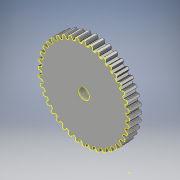
# Autodesk Inventor part: Engranaje_V_G_1
Saved by Autodesk Inventor 2017 (Build 210142000, 142)
## iProperties
Created: 2016-10-02
Part Number: Engranaje_V_G_1
Material: Generic
Document SubType Name: Modeling
Designer: CASA
Density: 1 g/cm^3
Appearance: Default
Author: CASA
Autodesk Inventor part; units mm, degrees
(part 1 of 3)
ref_plane "YZ Plane" through (0, 0, 0) normal (1, 0, 0) x (0, 1, 0)
ref_plane "XZ Plane" through (0, 0, 0) normal (0, 1, 0) x (-1, 0, 0)
ref_plane "XY Plane" through (0, 0, 0) normal (0, 0, 1) x (1, 0, 0)
sketch "Sketch1" plane through (0, 0, 0) normal (0, 1, 0) x (-1, 0, 0)
  line L0 (1.2517, 1.1017) -> (1.2466, 1.0629)
  line L1 (1.2466, 1.0629) -> (1.2316, 1.0267)
  line L2 (1.2316, 1.0267) -> (1.2078, 0.9957)
  line L3 (1.2078, 0.9957) -> (1.1767, 0.9718)
  line L4 (1.1767, 0.9718) -> (1.1405, 0.9568)
  line L5 (1.1405, 0.9568) -> (1.1017, 0.9517)
  line L6 (1.1017, 0.9517) -> (1.0629, 0.9568)
  line L7 (1.0629, 0.9568) -> (1.0267, 0.9718)
  line L8 (1.0267, 0.9718) -> (0.9956, 0.9956)
  line L9 (0.9956, 0.9956) -> (0.9718, 1.0267)
  line L10 (0.9718, 1.0267) -> (0.9568, 1.0629)
  line L11 (0.9568, 1.0629) -> (0.9517, 1.1017)
  line L12 (0.9517, 1.1017) -> (0.9568, 1.1405)
  line L13 (0.9568, 1.1405) -> (0.9718, 1.1767)
  line L14 (0.9718, 1.1767) -> (0.9956, 1.2078)
  line L15 (0.9956, 1.2078) -> (1.0267, 1.2316)
  line L16 (1.0267, 1.2316) -> (1.0629, 1.2466)
  line L17 (1.0629, 1.2466) -> (1.1017, 1.2517)
  line L18 (1.1017, 1.2517) -> (1.1405, 1.2466)
  line L19 (1.1405, 1.2466) -> (1.1767, 1.2316)
  line L20 (1.1767, 1.2316) -> (1.2078, 1.2078)
  line L21 (1.2078, 1.2078) -> (1.2316, 1.1767)
  line L22 (1.2316, 1.1767) -> (1.2466, 1.1405)
  line L23 (1.2466, 1.1405) -> (1.2517, 1.1017)
  line L24 (2.1254, 1.1532) -> (2.1288, 1.1525)
  line L25 (2.1288, 1.1525) -> (2.1355, 1.1511)
  line L26 (2.1355, 1.1511) -> (2.149, 1.1477)
  line L27 (2.149, 1.1477) -> (2.1625, 1.1437)
  line L28 (2.1625, 1.1437) -> (2.1761, 1.139)
  line L29 (2.1761, 1.139) -> (2.1896, 1.1339)
  line L30 (2.1896, 1.1339) -> (2.2031, 1.1282)
  line L31 (2.2031, 1.1282) -> (2.2031, 1.0756)
  line L32 (2.2031, 1.0756) -> (2.1896, 1.0699)
  line L33 (2.1896, 1.0699) -> (2.1761, 1.0647)
  line L34 (2.1761, 1.0647) -> (2.1626, 1.0601)
  line L35 (2.1626, 1.0601) -> (2.1491, 1.0561)
  line L36 (2.1491, 1.0561) -> (2.1356, 1.0527)
  line L37 (2.1356, 1.0527) -> (2.1288, 1.0513)
  line L38 (2.1288, 1.0513) -> (2.1254, 1.0506)
  line L39 (2.1254, 1.0506) -> (2.1221, 1.05)
  line L40 (2.1221, 1.05) -> (2.1176, 0.9935)
  line L41 (2.1176, 0.9935) -> (2.1209, 0.9923)
  line L42 (2.1209, 0.9923) -> (2.1241, 0.9912)
  line L43 (2.1241, 0.9912) -> (2.1305, 0.9887)
  line L44 (2.1305, 0.9887) -> (2.1433, 0.9832)
  line L45 (2.1433, 0.9832) -> (2.156, 0.9772)
  line L46 (2.156, 0.9772) -> (2.1687, 0.9705)
  line L47 (2.1687, 0.9705) -> (2.1812, 0.9633)
  line L48 (2.1812, 0.9633) -> (2.1936, 0.9556)
  line L49 (2.1936, 0.9556) -> (2.1854, 0.9035)
  line L50 (2.1854, 0.9035) -> (2.1712, 0.9)
  line L51 (2.1712, 0.9) -> (2.1571, 0.897)
  line L52 (2.1571, 0.897) -> (2.143, 0.8945)
  line L53 (2.143, 0.8945) -> (2.129, 0.8927)
  line L54 (2.129, 0.8927) -> (2.1151, 0.8914)
  line L55 (2.1151, 0.8914) -> (2.1083, 0.8911)
  line L56 (2.1083, 0.8911) -> (2.1048, 0.891)
  line L57 (2.1048, 0.891) -> (2.1014, 0.8909)
  line L58 (2.1014, 0.8909) -> (2.0882, 0.8357)
  line L59 (2.0882, 0.8357) -> (2.0912, 0.8341)
  line L60 (2.0912, 0.8341) -> (2.0942, 0.8325)
  line L61 (2.0942, 0.8325) -> (2.1002, 0.829)
  line L62 (2.1002, 0.829) -> (2.112, 0.8216)
  line L63 (2.112, 0.8216) -> (2.1236, 0.8136)
  line L64 (2.1236, 0.8136) -> (2.135, 0.8051)
  line L65 (2.135, 0.8051) -> (2.1462, 0.796)
  line L66 (2.1462, 0.796) -> (2.1573, 0.7864)
  line L67 (2.1573, 0.7864) -> (2.1411, 0.7364)
  line L68 (2.1411, 0.7364) -> (2.1265, 0.7351)
  line L69 (2.1265, 0.7351) -> (2.112, 0.7344)
  line L70 (2.112, 0.7344) -> (2.0978, 0.7342)
  line L71 (2.0978, 0.7342) -> (2.0837, 0.7345)
  line L72 (2.0837, 0.7345) -> (2.0698, 0.7355)
  line L73 (2.0698, 0.7355) -> (2.0629, 0.7362)
  line L74 (2.0629, 0.7362) -> (2.0595, 0.7366)
  line L75 (2.0595, 0.7366) -> (2.0561, 0.7371)
  line L76 (2.0561, 0.7371) -> (2.0344, 0.6847)
  line L77 (2.0344, 0.6847) -> (2.0371, 0.6826)
  line L78 (2.0371, 0.6826) -> (2.0398, 0.6805)
  line L79 (2.0398, 0.6805) -> (2.0452, 0.6762)
  line L80 (2.0452, 0.6762) -> (2.0557, 0.667)
  line L81 (2.0557, 0.667) -> (2.0659, 0.6573)
  line L82 (2.0659, 0.6573) -> (2.0759, 0.6471)
  line L83 (2.0759, 0.6471) -> (2.0856, 0.6363)
  line L84 (2.0856, 0.6363) -> (2.095, 0.6252)
  line L85 (2.095, 0.6252) -> (2.0711, 0.5783)
  line L86 (2.0711, 0.5783) -> (2.0565, 0.5794)
  line L87 (2.0565, 0.5794) -> (2.0421, 0.5809)
  line L88 (2.0421, 0.5809) -> (2.028, 0.5829)
  line L89 (2.028, 0.5829) -> (2.0141, 0.5855)
  line L90 (2.0141, 0.5855) -> (2.0006, 0.5886)
  line L91 (2.0006, 0.5886) -> (1.9939, 0.5903)
  line L92 (1.9939, 0.5903) -> (1.9906, 0.5913)
  line L93 (1.9906, 0.5913) -> (1.9873, 0.5923)
  line L94 (1.9873, 0.5923) -> (1.9577, 0.5439)
  line L95 (1.9577, 0.5439) -> (1.9601, 0.5415)
  line L96 (1.9601, 0.5415) -> (1.9624, 0.5389)
  line L97 (1.9624, 0.5389) -> (1.967, 0.5338)
  line L98 (1.967, 0.5338) -> (1.976, 0.5231)
  line L99 (1.976, 0.5231) -> (1.9845, 0.5119)
  line L100 (1.9845, 0.5119) -> (1.9928, 0.5003)
  line L101 (1.9928, 0.5003) -> (2.0006, 0.4882)
  line L102 (2.0006, 0.4882) -> (2.0082, 0.4756)
  line L103 (2.0082, 0.4756) -> (1.9773, 0.4331)
  line L104 (1.9773, 0.4331) -> (1.9631, 0.4364)
  line L105 (1.9631, 0.4364) -> (1.9491, 0.4402)
  line L106 (1.9491, 0.4402) -> (1.9355, 0.4444)
  line L107 (1.9355, 0.4444) -> (1.9221, 0.4491)
  line L108 (1.9221, 0.4491) -> (1.9092, 0.4543)
  line L109 (1.9092, 0.4543) -> (1.9029, 0.4571)
  line L110 (1.9029, 0.4571) -> (1.8998, 0.4585)
  line L111 (1.8998, 0.4585) -> (1.8968, 0.46)
  line L112 (1.8968, 0.46) -> (1.8599, 0.4169)
  line L113 (1.8599, 0.4169) -> (1.8619, 0.4141)
  line L114 (1.8619, 0.4141) -> (1.8638, 0.4112)
  line L115 (1.8638, 0.4112) -> (1.8675, 0.4054)
  line L116 (1.8675, 0.4054) -> (1.8747, 0.3935)
  line L117 (1.8747, 0.3935) -> (1.8814, 0.3811)
  line L118 (1.8814, 0.3811) -> (1.8877, 0.3683)
  line L119 (1.8877, 0.3683) -> (1.8936, 0.3551)
  line L120 (1.8936, 0.3551) -> (1.8991, 0.3415)
  line L121 (1.8991, 0.3415) -> (1.8619, 0.3043)
  line L122 (1.8619, 0.3043) -> (1.8484, 0.3099)
  line L123 (1.8484, 0.3099) -> (1.8352, 0.3158)
  line L124 (1.8352, 0.3158) -> (1.8224, 0.3221)
  line L125 (1.8224, 0.3221) -> (1.81, 0.3288)
  line L126 (1.81, 0.3288) -> (1.798, 0.3359)
  line L127 (1.798, 0.3359) -> (1.7922, 0.3397)
  line L128 (1.7922, 0.3397) -> (1.7894, 0.3416)
  line L129 (1.7894, 0.3416) -> (1.7866, 0.3436)
  line L130 (1.7866, 0.3436) -> (1.7434, 0.3067)
  line L131 (1.7434, 0.3067) -> (1.7449, 0.3036)
  line L132 (1.7449, 0.3036) -> (1.7464, 0.3005)
  line L133 (1.7464, 0.3005) -> (1.7492, 0.2942)
  line L134 (1.7492, 0.2942) -> (1.7544, 0.2813)
  line L135 (1.7544, 0.2813) -> (1.7591, 0.268)
  line L136 (1.7591, 0.268) -> (1.7633, 0.2544)
  line L137 (1.7633, 0.2544) -> (1.7671, 0.2404)
  line L138 (1.7671, 0.2404) -> (1.7704, 0.2261)
  line L139 (1.7704, 0.2261) -> (1.7278, 0.1952)
  line L140 (1.7278, 0.1952) -> (1.7153, 0.2028)
  line L141 (1.7153, 0.2028) -> (1.7032, 0.2107)
  line L142 (1.7032, 0.2107) -> (1.6915, 0.2189)
  line L143 (1.6915, 0.2189) -> (1.6803, 0.2275)
  line L144 (1.6803, 0.2275) -> (1.6696, 0.2364)
  line L145 (1.6696, 0.2364) -> (1.6645, 0.241)
  line L146 (1.6645, 0.241) -> (1.662, 0.2434)
  line L147 (1.662, 0.2434) -> (1.6596, 0.2458)
  line L148 (1.6596, 0.2458) -> (1.6112, 0.2161)
  line L149 (1.6112, 0.2161) -> (1.6122, 0.2128)
  line L150 (1.6122, 0.2128) -> (1.6131, 0.2095)
  line L151 (1.6131, 0.2095) -> (1.6149, 0.2029)
  line L152 (1.6149, 0.2029) -> (1.618, 0.1893)
  line L153 (1.618, 0.1893) -> (1.6206, 0.1754)
  line L154 (1.6206, 0.1754) -> (1.6226, 0.1613)
  line L155 (1.6226, 0.1613) -> (1.6241, 0.1469)
  line L156 (1.6241, 0.1469) -> (1.6252, 0.1323)
  line L157 (1.6252, 0.1323) -> (1.5783, 0.1084)
  line L158 (1.5783, 0.1084) -> (1.5671, 0.1179)
  line L159 (1.5671, 0.1179) -> (1.5564, 0.1276)
  line L160 (1.5564, 0.1276) -> (1.5462, 0.1375)
  line L161 (1.5462, 0.1375) -> (1.5364, 0.1477)
  line L162 (1.5364, 0.1477) -> (1.5273, 0.1582)
  line L163 (1.5273, 0.1582) -> (1.5229, 0.1636)
  line L164 (1.5229, 0.1636) -> (1.5208, 0.1663)
  line L165 (1.5208, 0.1663) -> (1.5188, 0.169)
  line L166 (1.5188, 0.169) -> (1.4663, 0.1473)
  line L167 (1.4663, 0.1473) -> (1.4668, 0.1439)
  line L168 (1.4668, 0.1439) -> (1.4673, 0.1405)
  line L169 (1.4673, 0.1405) -> (1.468, 0.1337)
  line L170 (1.468, 0.1337) -> (1.4689, 0.1198)
  line L171 (1.4689, 0.1198) -> (1.4693, 0.1057)
  line L172 (1.4693, 0.1057) -> (1.469, 0.0914)
  line L173 (1.469, 0.0914) -> (1.4683, 0.077)
  line L174 (1.4683, 0.077) -> (1.4671, 0.0624)
  line L175 (1.4671, 0.0624) -> (1.4171, 0.0461)
  line L176 (1.4171, 0.0461) -> (1.4075, 0.0572)
  line L177 (1.4075, 0.0572) -> (1.3984, 0.0684)
  line L178 (1.3984, 0.0684) -> (1.3898, 0.0799)
  line L179 (1.3898, 0.0799) -> (1.3818, 0.0915)
  line L180 (1.3818, 0.0915) -> (1.3744, 0.1033)
  line L181 (1.3744, 0.1033) -> (1.371, 0.1092)
  line L182 (1.371, 0.1092) -> (1.3693, 0.1123)
  line L183 (1.3693, 0.1123) -> (1.3677, 0.1153)
  line L184 (1.3677, 0.1153) -> (1.3126, 0.102)
  line L185 (1.3126, 0.102) -> (1.3125, 0.0986)
  line L186 (1.3125, 0.0986) -> (1.3124, 0.0952)
  line L187 (1.3124, 0.0952) -> (1.312, 0.0883)
  line L188 (1.312, 0.0883) -> (1.3108, 0.0744)
  line L189 (1.3108, 0.0744) -> (1.3089, 0.0604)
  line L190 (1.3089, 0.0604) -> (1.3065, 0.0464)
  line L191 (1.3065, 0.0464) -> (1.3035, 0.0322)
  line L192 (1.3035, 0.0322) -> (1.3, 0.018)
  line L193 (1.3, 0.018) -> (1.248, 0.0098)
  line L194 (1.248, 0.0098) -> (1.2403, 0.0222)
  line L195 (1.2403, 0.0222) -> (1.2331, 0.0348)
  line L196 (1.2331, 0.0348) -> (1.2264, 0.0474)
  line L197 (1.2264, 0.0474) -> (1.2203, 0.0601)
  line L198 (1.2203, 0.0601) -> (1.2149, 0.0729)
  line L199 (1.2149, 0.0729) -> (1.2124, 0.0793)
  line L200 (1.2124, 0.0793) -> (1.2112, 0.0826)
  line L201 (1.2112, 0.0826) -> (1.2101, 0.0858)
  line L202 (1.2101, 0.0858) -> (1.1536, 0.0814)
  line L203 (1.1536, 0.0814) -> (1.153, 0.078)
  line L204 (1.153, 0.078) -> (1.1523, 0.0746)
  line L205 (1.1523, 0.0746) -> (1.1509, 0.0679)
  line L206 (1.1509, 0.0679) -> (1.1475, 0.0544)
  line L207 (1.1475, 0.0544) -> (1.1435, 0.0409)
  line L208 (1.1435, 0.0409) -> (1.1389, 0.0273)
  line L209 (1.1389, 0.0273) -> (1.1337, 0.0138)
  line L210 (1.1337, 0.0138) -> (1.128, 0.0003)
  line L211 (1.128, 0.0003) -> (1.0754, 0.0003)
  line L212 (1.0754, 0.0003) -> (1.0697, 0.0138)
  line L213 (1.0697, 0.0138) -> (1.0646, 0.0273)
  line L214 (1.0646, 0.0273) -> (1.06, 0.0409)
  line L215 (1.06, 0.0409) -> (1.0559, 0.0544)
  line L216 (1.0559, 0.0544) -> (1.0525, 0.0679)
  line L217 (1.0525, 0.0679) -> (1.0511, 0.0746)
  line L218 (1.0511, 0.0746) -> (1.0505, 0.078)
  line L219 (1.0505, 0.078) -> (1.0499, 0.0814)
  line L220 (1.0499, 0.0814) -> (0.9933, 0.0858)
  line L221 (0.9933, 0.0858) -> (0.9922, 0.0826)
  line L222 (0.9922, 0.0826) -> (0.991, 0.0793)
  line L223 (0.991, 0.0793) -> (0.9886, 0.0729)
  line L224 (0.9886, 0.0729) -> (0.9831, 0.0601)
  line L225 (0.9831, 0.0601) -> (0.977, 0.0474)
  line L226 (0.977, 0.0474) -> (0.9703, 0.0348)
  line L227 (0.9703, 0.0348) -> (0.9631, 0.0222)
  line L228 (0.9631, 0.0222) -> (0.9554, 0.0098)
  line L229 (0.9554, 0.0098) -> (0.9034, 0.018)
  line L230 (0.9034, 0.018) -> (0.9, 0.0322)
  line L231 (0.9, 0.0322) -> (0.897, 0.0464)
  line L232 (0.897, 0.0464) -> (0.8945, 0.0604)
  line L233 (0.8945, 0.0604) -> (0.8927, 0.0744)
  line L234 (0.8927, 0.0744) -> (0.8914, 0.0883)
  line L235 (0.8914, 0.0883) -> (0.8911, 0.0952)
  line L236 (0.8911, 0.0952) -> (0.891, 0.0986)
  line L237 (0.891, 0.0986) -> (0.8909, 0.102)
  line L238 (0.8909, 0.102) -> (0.8357, 0.1153)
  line L239 (0.8357, 0.1153) -> (0.8341, 0.1123)
  line L240 (0.8341, 0.1123) -> (0.8325, 0.1093)
  line L241 (0.8325, 0.1093) -> (0.829, 0.1033)
  line L242 (0.829, 0.1033) -> (0.8216, 0.0915)
  line L243 (0.8216, 0.0915) -> (0.8136, 0.0799)
  line L244 (0.8136, 0.0799) -> (0.805, 0.0685)
  line L245 (0.805, 0.0685) -> (0.796, 0.0572)
  line L246 (0.796, 0.0572) -> (0.7864, 0.0461)
  line L247 (0.7864, 0.0461) -> (0.7364, 0.0624)
  line L248 (0.7364, 0.0624) -> (0.7351, 0.077)
  line L249 (0.7351, 0.077) -> (0.7344, 0.0914)
  line L250 (0.7344, 0.0914) -> (0.7342, 0.1057)
  line L251 (0.7342, 0.1057) -> (0.7345, 0.1198)
  line L252 (0.7345, 0.1198) -> (0.7355, 0.1337)
  line L253 (0.7355, 0.1337) -> (0.7362, 0.1405)
  line L254 (0.7362, 0.1405) -> (0.7366, 0.1439)
  line L255 (0.7366, 0.1439) -> (0.7371, 0.1473)
  line L256 (0.7371, 0.1473) -> (0.6847, 0.169)
  line L257 (0.6847, 0.169) -> (0.6826, 0.1663)
  line L258 (0.6826, 0.1663) -> (0.6805, 0.1636)
  line L259 (0.6805, 0.1636) -> (0.6762, 0.1582)
  line L260 (0.6762, 0.1582) -> (0.667, 0.1477)
  line L261 (0.667, 0.1477) -> (0.6573, 0.1375)
  line L262 (0.6573, 0.1375) -> (0.647, 0.1276)
  line L263 (0.647, 0.1276) -> (0.6363, 0.1179)
  line L264 (0.6363, 0.1179) -> (0.6251, 0.1084)
  line L265 (0.6251, 0.1084) -> (0.5783, 0.1323)
  line L266 (0.5783, 0.1323) -> (0.5793, 0.1469)
  line L267 (0.5793, 0.1469) -> (0.5809, 0.1613)
  line L268 (0.5809, 0.1613) -> (0.5829, 0.1754)
  line L269 (0.5829, 0.1754) -> (0.5854, 0.1893)
  line L270 (0.5854, 0.1893) -> (0.5885, 0.2029)
  line L271 (0.5885, 0.2029) -> (0.5903, 0.2095)
  line L272 (0.5903, 0.2095) -> (0.5913, 0.2128)
  line L273 (0.5913, 0.2128) -> (0.5923, 0.2161)
  line L274 (0.5923, 0.2161) -> (0.5439, 0.2457)
  line L275 (0.5439, 0.2457) -> (0.5414, 0.2434)
  line L276 (0.5414, 0.2434) -> (0.5389, 0.241)
  line L277 (0.5389, 0.241) -> (0.5338, 0.2364)
  line L278 (0.5338, 0.2364) -> (0.5231, 0.2275)
  line L279 (0.5231, 0.2275) -> (0.5119, 0.2189)
  line L280 (0.5119, 0.2189) -> (0.5002, 0.2107)
  line L281 (0.5002, 0.2107) -> (0.4881, 0.2028)
  line L282 (0.4881, 0.2028) -> (0.4756, 0.1952)
  line L283 (0.4756, 0.1952) -> (0.4331, 0.2261)
  line L284 (0.4331, 0.2261) -> (0.4364, 0.2404)
  line L285 (0.4364, 0.2404) -> (0.4402, 0.2543)
  line L286 (0.4402, 0.2543) -> (0.4444, 0.268)
  line L287 (0.4444, 0.268) -> (0.449, 0.2813)
  line L288 (0.449, 0.2813) -> (0.4542, 0.2942)
  line L289 (0.4542, 0.2942) -> (0.457, 0.3005)
  line L290 (0.457, 0.3005) -> (0.4585, 0.3036)
  line L291 (0.4585, 0.3036) -> (0.46, 0.3067)
  line L292 (0.46, 0.3067) -> (0.4168, 0.3435)
  line L293 (0.4168, 0.3435) -> (0.414, 0.3416)
  line L294 (0.414, 0.3416) -> (0.4112, 0.3396)
  line L295 (0.4112, 0.3396) -> (0.4054, 0.3359)
  line L296 (0.4054, 0.3359) -> (0.3935, 0.3287)
  line L297 (0.3935, 0.3287) -> (0.3811, 0.322)
  line L298 (0.3811, 0.322) -> (0.3683, 0.3157)
  line L299 (0.3683, 0.3157) -> (0.3551, 0.3098)
  line L300 (0.3551, 0.3098) -> (0.3415, 0.3043)
  line L301 (0.3415, 0.3043) -> (0.3043, 0.3415)
  line L302 (0.3043, 0.3415) -> (0.3098, 0.3551)
  line L303 (0.3098, 0.3551) -> (0.3157, 0.3683)
  line L304 (0.3157, 0.3683) -> (0.322, 0.3811)
  line L305 (0.322, 0.3811) -> (0.3287, 0.3935)
  line L306 (0.3287, 0.3935) -> (0.3359, 0.4054)
  line L307 (0.3359, 0.4054) -> (0.3396, 0.4112)
  line L308 (0.3396, 0.4112) -> (0.3416, 0.4141)
  line L309 (0.3416, 0.4141) -> (0.3435, 0.4169)
  line L310 (0.3435, 0.4169) -> (0.3067, 0.46)
  line L311 (0.3067, 0.46) -> (0.3036, 0.4585)
  line L312 (0.3036, 0.4585) -> (0.3005, 0.457)
  line L313 (0.3005, 0.457) -> (0.2942, 0.4542)
  line L314 (0.2942, 0.4542) -> (0.2813, 0.449)
  line L315 (0.2813, 0.449) -> (0.268, 0.4444)
  line L316 (0.268, 0.4444) -> (0.2543, 0.4402)
  line L317 (0.2543, 0.4402) -> (0.2404, 0.4364)
  line L318 (0.2404, 0.4364) -> (0.2261, 0.4331)
  line L319 (0.2261, 0.4331) -> (0.1952, 0.4756)
  line L320 (0.1952, 0.4756) -> (0.2028, 0.4881)
  line L321 (0.2028, 0.4881) -> (0.2107, 0.5002)
  line L322 (0.2107, 0.5002) -> (0.2189, 0.5119)
  line L323 (0.2189, 0.5119) -> (0.2275, 0.5231)
  line L324 (0.2275, 0.5231) -> (0.2364, 0.5338)
  line L325 (0.2364, 0.5338) -> (0.241, 0.5389)
  line L326 (0.241, 0.5389) -> (0.2434, 0.5414)
  line L327 (0.2434, 0.5414) -> (0.2457, 0.5439)
  line L328 (0.2457, 0.5439) -> (0.2161, 0.5923)
  line L329 (0.2161, 0.5923) -> (0.2128, 0.5913)
  line L330 (0.2128, 0.5913) -> (0.2095, 0.5903)
  line L331 (0.2095, 0.5903) -> (0.2029, 0.5885)
  line L332 (0.2029, 0.5885) -> (0.1893, 0.5854)
  line L333 (0.1893, 0.5854) -> (0.1754, 0.5829)
  line L334 (0.1754, 0.5829) -> (0.1613, 0.5809)
  line L335 (0.1613, 0.5809) -> (0.1469, 0.5793)
  line L336 (0.1469, 0.5793) -> (0.1323, 0.5782)
  line L337 (0.1323, 0.5782) -> (0.1084, 0.6251)
  line L338 (0.1084, 0.6251) -> (0.1179, 0.6363)
  line L339 (0.1179, 0.6363) -> (0.1276, 0.647)
  line L340 (0.1276, 0.647) -> (0.1375, 0.6573)
  line L341 (0.1375, 0.6573) -> (0.1477, 0.667)
  line L342 (0.1477, 0.667) -> (0.1582, 0.6762)
  line L343 (0.1582, 0.6762) -> (0.1636, 0.6805)
  line L344 (0.1636, 0.6805) -> (0.1663, 0.6826)
  line L345 (0.1663, 0.6826) -> (0.169, 0.6847)
  line L346 (0.169, 0.6847) -> (0.1473, 0.7371)
  line L347 (0.1473, 0.7371) -> (0.1439, 0.7366)
  line L348 (0.1439, 0.7366) -> (0.1405, 0.7362)
  line L349 (0.1405, 0.7362) -> (0.1336, 0.7355)
  line L350 (0.1336, 0.7355) -> (0.1197, 0.7345)
  line L351 (0.1197, 0.7345) -> (0.1056, 0.7342)
  line L352 (0.1056, 0.7342) -> (0.0914, 0.7344)
  line L353 (0.0914, 0.7344) -> (0.0769, 0.7351)
  line L354 (0.0769, 0.7351) -> (0.0624, 0.7363)
  line L355 (0.0624, 0.7363) -> (0.0461, 0.7864)
  line L356 (0.0461, 0.7864) -> (0.0572, 0.7959)
  line L357 (0.0572, 0.7959) -> (0.0684, 0.805)
  line L358 (0.0684, 0.805) -> (0.0799, 0.8136)
  line L359 (0.0799, 0.8136) -> (0.0915, 0.8216)
  line L360 (0.0915, 0.8216) -> (0.1033, 0.829)
  line L361 (0.1033, 0.829) -> (0.1092, 0.8324)
  line L362 (0.1092, 0.8324) -> (0.1122, 0.8341)
  line L363 (0.1122, 0.8341) -> (0.1153, 0.8357)
  line L364 (0.1153, 0.8357) -> (0.102, 0.8909)
  line L365 (0.102, 0.8909) -> (0.0986, 0.8909)
  line L366 (0.0986, 0.8909) -> (0.0952, 0.891)
  line L367 (0.0952, 0.891) -> (0.0883, 0.8914)
  line L368 (0.0883, 0.8914) -> (0.0744, 0.8926)
  line L369 (0.0744, 0.8926) -> (0.0604, 0.8945)
  line L370 (0.0604, 0.8945) -> (0.0464, 0.897)
  line L371 (0.0464, 0.897) -> (0.0322, 0.8999)
  line L372 (0.0322, 0.8999) -> (0.018, 0.9034)
  line L373 (0.018, 0.9034) -> (0.0098, 0.9554)
  line L374 (0.0098, 0.9554) -> (0.0222, 0.9631)
  line L375 (0.0222, 0.9631) -> (0.0347, 0.9703)
  line L376 (0.0347, 0.9703) -> (0.0474, 0.977)
  line L377 (0.0474, 0.977) -> (0.0601, 0.9831)
  line L378 (0.0601, 0.9831) -> (0.0729, 0.9885)
  line L379 (0.0729, 0.9885) -> (0.0793, 0.991)
  line L380 (0.0793, 0.991) -> (0.0825, 0.9922)
  line L381 (0.0825, 0.9922) -> (0.0858, 0.9933)
  line L382 (0.0858, 0.9933) -> (0.0813, 1.0499)
  line L383 (0.0813, 1.0499) -> (0.078, 1.0505)
  line L384 (0.078, 1.0505) -> (0.0746, 1.0511)
  line L385 (0.0746, 1.0511) -> (0.0678, 1.0525)
  line L386 (0.0678, 1.0525) -> (0.0543, 1.0559)
  line L387 (0.0543, 1.0559) -> (0.0408, 1.06)
  line L388 (0.0408, 1.06) -> (0.0273, 1.0646)
  line L389 (0.0273, 1.0646) -> (0.0138, 1.0697)
  line L390 (0.0138, 1.0697) -> (0.0003, 1.0754)
  line L391 (0.0003, 1.0754) -> (0.0003, 1.128)
  line L392 (0.0003, 1.128) -> (0.0138, 1.1337)
  line L393 (0.0138, 1.1337) -> (0.0273, 1.1388)
  line L394 (0.0273, 1.1388) -> (0.0408, 1.1435)
  line L395 (0.0408, 1.1435) -> (0.0543, 1.1475)
  line L396 (0.0543, 1.1475) -> (0.0678, 1.1509)
  line L397 (0.0678, 1.1509) -> (0.0746, 1.1523)
  line L398 (0.0746, 1.1523) -> (0.078, 1.153)
  line L399 (0.078, 1.153) -> (0.0813, 1.1536)
  line L400 (0.0813, 1.1536) -> (0.0858, 1.2101)
  line L401 (0.0858, 1.2101) -> (0.0825, 1.2112)
  line L402 (0.0825, 1.2112) -> (0.0793, 1.2124)
  line L403 (0.0793, 1.2124) -> (0.0729, 1.2149)
  line L404 (0.0729, 1.2149) -> (0.0601, 1.2203)
  line L405 (0.0601, 1.2203) -> (0.0474, 1.2264)
  line L406 (0.0474, 1.2264) -> (0.0347, 1.2331)
  line L407 (0.0347, 1.2331) -> (0.0222, 1.2403)
  line L408 (0.0222, 1.2403) -> (0.0098, 1.248)
  line L409 (0.0098, 1.248) -> (0.018, 1.3)
  line L410 (0.018, 1.3) -> (0.0322, 1.3035)
  line L411 (0.0322, 1.3035) -> (0.0464, 1.3065)
  line L412 (0.0464, 1.3065) -> (0.0604, 1.3089)
  line L413 (0.0604, 1.3089) -> (0.0744, 1.3108)
  line L414 (0.0744, 1.3108) -> (0.0883, 1.312)
  line L415 (0.0883, 1.312) -> (0.0952, 1.3124)
  line L416 (0.0952, 1.3124) -> (0.0986, 1.3125)
  line L417 (0.0986, 1.3125) -> (0.102, 1.3125)
  line L418 (0.102, 1.3125) -> (0.1153, 1.3677)
  line L419 (0.1153, 1.3677) -> (0.1122, 1.3693)
  line L420 (0.1122, 1.3693) -> (0.1092, 1.371)
  line L421 (0.1092, 1.371) -> (0.1033, 1.3744)
  line L422 (0.1033, 1.3744) -> (0.0915, 1.3818)
  line L423 (0.0915, 1.3818) -> (0.0799, 1.3898)
  line L424 (0.0799, 1.3898) -> (0.0684, 1.3984)
  line L425 (0.0684, 1.3984) -> (0.0572, 1.4075)
  line L426 (0.0572, 1.4075) -> (0.0461, 1.417)
  line L427 (0.0461, 1.417) -> (0.0624, 1.4671)
  line L428 (0.0624, 1.4671) -> (0.0769, 1.4683)
  line L429 (0.0769, 1.4683) -> (0.0914, 1.469)
  line L430 (0.0914, 1.469) -> (0.1056, 1.4692)
  line L431 (0.1056, 1.4692) -> (0.1197, 1.4689)
  line L432 (0.1197, 1.4689) -> (0.1336, 1.468)
  line L433 (0.1336, 1.468) -> (0.1405, 1.4672)
  line L434 (0.1405, 1.4672) -> (0.1439, 1.4668)
  line L435 (0.1439, 1.4668) -> (0.1473, 1.4663)
  line L436 (0.1473, 1.4663) -> (0.169, 1.5188)
  line L437 (0.169, 1.5188) -> (0.1663, 1.5208)
  line L438 (0.1663, 1.5208) -> (0.1636, 1.5229)
  line L439 (0.1636, 1.5229) -> (0.1582, 1.5273)
  line L440 (0.1582, 1.5273) -> (0.1477, 1.5364)
  line L441 (0.1477, 1.5364) -> (0.1375, 1.5461)
  line L442 (0.1375, 1.5461) -> (0.1275, 1.5564)
  line L443 (0.1275, 1.5564) -> (0.1179, 1.5671)
  line L444 (0.1179, 1.5671) -> (0.1084, 1.5783)
  line L445 (0.1084, 1.5783) -> (0.1323, 1.6252)
  line L446 (0.1323, 1.6252) -> (0.1469, 1.6241)
  line L447 (0.1469, 1.6241) -> (0.1613, 1.6226)
  line L448 (0.1613, 1.6226) -> (0.1754, 1.6205)
  line L449 (0.1754, 1.6205) -> (0.1893, 1.618)
  line L450 (0.1893, 1.618) -> (0.2028, 1.6149)
  line L451 (0.2028, 1.6149) -> (0.2095, 1.6131)
  line L452 (0.2095, 1.6131) -> (0.2128, 1.6122)
  line L453 (0.2128, 1.6122) -> (0.2161, 1.6112)
  line L454 (0.2161, 1.6112) -> (0.2457, 1.6595)
  line L455 (0.2457, 1.6595) -> (0.2433, 1.662)
  line L456 (0.2433, 1.662) -> (0.241, 1.6645)
  line L457 (0.241, 1.6645) -> (0.2364, 1.6696)
  line L458 (0.2364, 1.6696) -> (0.2274, 1.6803)
  line L459 (0.2274, 1.6803) -> (0.2189, 1.6915)
  line L460 (0.2189, 1.6915) -> (0.2106, 1.7032)
  line L461 (0.2106, 1.7032) -> (0.2028, 1.7153)
  line L462 (0.2028, 1.7153) -> (0.1952, 1.7278)
  line L463 (0.1952, 1.7278) -> (0.2261, 1.7704)
  line L464 (0.2261, 1.7704) -> (0.2403, 1.767)
  line L465 (0.2403, 1.767) -> (0.2543, 1.7633)
  line L466 (0.2543, 1.7633) -> (0.268, 1.7591)
  line L467 (0.268, 1.7591) -> (0.2813, 1.7544)
  line L468 (0.2813, 1.7544) -> (0.2942, 1.7492)
  line L469 (0.2942, 1.7492) -> (0.3005, 1.7464)
  line L470 (0.3005, 1.7464) -> (0.3036, 1.7449)
  line L471 (0.3036, 1.7449) -> (0.3067, 1.7434)
  line L472 (0.3067, 1.7434) -> (0.3435, 1.7866)
  line L473 (0.3435, 1.7866) -> (0.3415, 1.7894)
  line L474 (0.3415, 1.7894) -> (0.3396, 1.7922)
  line L475 (0.3396, 1.7922) -> (0.3358, 1.798)
  line L476 (0.3358, 1.798) -> (0.3287, 1.8099)
  line L477 (0.3287, 1.8099) -> (0.322, 1.8224)
  line L478 (0.322, 1.8224) -> (0.3157, 1.8352)
  line L479 (0.3157, 1.8352) -> (0.3098, 1.8484)
  line L480 (0.3098, 1.8484) -> (0.3043, 1.8619)
  line L481 (0.3043, 1.8619) -> (0.3415, 1.8991)
  line L482 (0.3415, 1.8991) -> (0.355, 1.8936)
  line L483 (0.355, 1.8936) -> (0.3682, 1.8877)
  line L484 (0.3682, 1.8877) -> (0.381, 1.8814)
  line L485 (0.381, 1.8814) -> (0.3934, 1.8747)
  line L486 (0.3934, 1.8747) -> (0.4054, 1.8676)
  line L487 (0.4054, 1.8676) -> (0.4112, 1.8638)
  line L488 (0.4112, 1.8638) -> (0.414, 1.8619)
  line L489 (0.414, 1.8619) -> (0.4168, 1.8599)
  line L490 (0.4168, 1.8599) -> (0.46, 1.8968)
  line L491 (0.46, 1.8968) -> (0.4585, 1.8998)
  line L492 (0.4585, 1.8998) -> (0.457, 1.9029)
  line L493 (0.457, 1.9029) -> (0.4542, 1.9092)
  line L494 (0.4542, 1.9092) -> (0.449, 1.9222)
  line L495 (0.449, 1.9222) -> (0.4443, 1.9355)
  line L496 (0.4443, 1.9355) -> (0.4401, 1.9491)
  line L497 (0.4401, 1.9491) -> (0.4363, 1.9631)
  line L498 (0.4363, 1.9631) -> (0.433, 1.9773)
  line L499 (0.433, 1.9773) -> (0.4756, 2.0082)
  line L500 (0.4756, 2.0082) -> (0.4881, 2.0007)
  line L501 (0.4881, 2.0007) -> (0.5002, 1.9928)
  line L502 (0.5002, 1.9928) -> (0.5119, 1.9845)
  line L503 (0.5119, 1.9845) -> (0.5231, 1.976)
  line L504 (0.5231, 1.976) -> (0.5338, 1.967)
  line L505 (0.5338, 1.967) -> (0.5389, 1.9624)
  line L506 (0.5389, 1.9624) -> (0.5414, 1.9601)
  line L507 (0.5414, 1.9601) -> (0.5438, 1.9577)
  line L508 (0.5438, 1.9577) -> (0.5922, 1.9874)
  line L509 (0.5922, 1.9874) -> (0.5912, 1.9906)
  line L510 (0.5912, 1.9906) -> (0.5903, 1.9939)
  line L511 (0.5903, 1.9939) -> (0.5885, 2.0006)
  line L512 (0.5885, 2.0006) -> (0.5854, 2.0142)
  line L513 (0.5854, 2.0142) -> (0.5828, 2.028)
  line L514 (0.5828, 2.028) -> (0.5808, 2.0422)
  line L515 (0.5808, 2.0422) -> (0.5793, 2.0565)
  line L516 (0.5793, 2.0565) -> (0.5782, 2.0711)
  line L517 (0.5782, 2.0711) -> (0.6251, 2.095)
  line L518 (0.6251, 2.095) -> (0.6363, 2.0856)
  line L519 (0.6363, 2.0856) -> (0.647, 2.0759)
  line L520 (0.647, 2.0759) -> (0.6572, 2.0659)
  line L521 (0.6572, 2.0659) -> (0.667, 2.0557)
  line L522 (0.667, 2.0557) -> (0.6761, 2.0452)
  line L523 (0.6761, 2.0452) -> (0.6805, 2.0399)
  line L524 (0.6805, 2.0399) -> (0.6826, 2.0372)
  line L525 (0.6826, 2.0372) -> (0.6846, 2.0344)
  line L526 (0.6846, 2.0344) -> (0.737, 2.0562)
  line L527 (0.737, 2.0562) -> (0.7366, 2.0595)
  line L528 (0.7366, 2.0595) -> (0.7361, 2.0629)
  line L529 (0.7361, 2.0629) -> (0.7354, 2.0698)
  line L530 (0.7354, 2.0698) -> (0.7345, 2.0837)
  line L531 (0.7345, 2.0837) -> (0.7341, 2.0978)
  line L532 (0.7341, 2.0978) -> (0.7343, 2.1121)
  line L533 (0.7343, 2.1121) -> (0.7351, 2.1265)
  line L534 (0.7351, 2.1265) -> (0.7363, 2.1411)
  line L535 (0.7363, 2.1411) -> (0.7863, 2.1573)
  line L536 (0.7863, 2.1573) -> (0.7959, 2.1463)
  line L537 (0.7959, 2.1463) -> (0.805, 2.135)
  line L538 (0.805, 2.135) -> (0.8135, 2.1236)
  line L539 (0.8135, 2.1236) -> (0.8215, 2.112)
  line L540 (0.8215, 2.112) -> (0.8289, 2.1002)
  line L541 (0.8289, 2.1002) -> (0.8324, 2.0942)
  line L542 (0.8324, 2.0942) -> (0.8341, 2.0912)
  line L543 (0.8341, 2.0912) -> (0.8357, 2.0882)
  line L544 (0.8357, 2.0882) -> (0.8908, 2.1014)
  line L545 (0.8908, 2.1014) -> (0.8909, 2.1049)
  line L546 (0.8909, 2.1049) -> (0.891, 2.1083)
  line L547 (0.891, 2.1083) -> (0.8914, 2.1152)
  line L548 (0.8914, 2.1152) -> (0.8926, 2.129)
  line L549 (0.8926, 2.129) -> (0.8945, 2.143)
  line L550 (0.8945, 2.143) -> (0.8969, 2.1571)
  line L551 (0.8969, 2.1571) -> (0.8999, 2.1712)
  line L552 (0.8999, 2.1712) -> (0.9034, 2.1855)
  line L553 (0.9034, 2.1855) -> (0.9553, 2.1937)
  line L554 (0.9553, 2.1937) -> (0.9631, 2.1812)
  line L555 (0.9631, 2.1812) -> (0.9703, 2.1687)
  line L556 (0.9703, 2.1687) -> (0.9769, 2.1561)
  line L557 (0.9769, 2.1561) -> (0.983, 2.1434)
  line L558 (0.983, 2.1434) -> (0.9885, 2.1306)
  line L559 (0.9885, 2.1306) -> (0.991, 2.1241)
  line L560 (0.991, 2.1241) -> (0.9921, 2.1209)
  line L561 (0.9921, 2.1209) -> (0.9932, 2.1177)
  line L562 (0.9932, 2.1177) -> (1.0498, 2.1221)
  line L563 (1.0498, 2.1221) -> (1.0504, 2.1255)
  line L564 (1.0504, 2.1255) -> (1.0511, 2.1289)
  line L565 (1.0511, 2.1289) -> (1.0525, 2.1356)
  line L566 (1.0525, 2.1356) -> (1.0559, 2.1491)
  line L567 (1.0559, 2.1491) -> (1.0599, 2.1626)
  line L568 (1.0599, 2.1626) -> (1.0645, 2.1761)
  line L569 (1.0645, 2.1761) -> (1.0697, 2.1896)
  line L570 (1.0697, 2.1896) -> (1.0754, 2.2031)
  line L571 (1.0754, 2.2031) -> (1.128, 2.2031)
  line L572 (1.128, 2.2031) -> (1.1336, 2.1896)
  line L573 (1.1336, 2.1896) -> (1.1388, 2.1761)
  line L574 (1.1388, 2.1761) -> (1.1434, 2.1626)
  line L575 (1.1434, 2.1626) -> (1.1474, 2.1491)
  line L576 (1.1474, 2.1491) -> (1.1508, 2.1356)
  line L577 (1.1508, 2.1356) -> (1.1523, 2.1289)
  line L578 (1.1523, 2.1289) -> (1.1529, 2.1255)
  line L579 (1.1529, 2.1255) -> (1.1535, 2.1221)
  line L580 (1.1535, 2.1221) -> (1.2101, 2.1177)
  line L581 (1.2101, 2.1177) -> (1.2112, 2.1209)
  line L582 (1.2112, 2.1209) -> (1.2124, 2.1241)
  line L583 (1.2124, 2.1241) -> (1.2148, 2.1306)
  line L584 (1.2148, 2.1306) -> (1.2203, 2.1434)
  line L585 (1.2203, 2.1434) -> (1.2264, 2.1561)
  line L586 (1.2264, 2.1561) -> (1.2331, 2.1687)
  line L587 (1.2331, 2.1687) -> (1.2403, 2.1812)
  line L588 (1.2403, 2.1812) -> (1.248, 2.1937)
  line L589 (1.248, 2.1937) -> (1.2999, 2.1855)
  line L590 (1.2999, 2.1855) -> (1.3034, 2.1712)
  line L591 (1.3034, 2.1712) -> (1.3064, 2.1571)
  line L592 (1.3064, 2.1571) -> (1.3089, 2.143)
  line L593 (1.3089, 2.143) -> (1.3107, 2.129)
  line L594 (1.3107, 2.129) -> (1.312, 2.1152)
  line L595 (1.312, 2.1152) -> (1.3123, 2.1083)
  line L596 (1.3123, 2.1083) -> (1.3124, 2.1049)
  line L597 (1.3124, 2.1049) -> (1.3125, 2.1014)
  line L598 (1.3125, 2.1014) -> (1.3677, 2.0882)
  line L599 (1.3677, 2.0882) -> (1.3693, 2.0912)
  line L600 (1.3693, 2.0912) -> (1.3709, 2.0942)
  line L601 (1.3709, 2.0942) -> (1.3744, 2.1002)
  line L602 (1.3744, 2.1002) -> (1.3818, 2.112)
  line L603 (1.3818, 2.112) -> (1.3898, 2.1236)
  line L604 (1.3898, 2.1236) -> (1.3983, 2.135)
  line L605 (1.3983, 2.135) -> (1.4074, 2.1463)
  line L606 (1.4074, 2.1463) -> (1.417, 2.1573)
  line L607 (1.417, 2.1573) -> (1.467, 2.1411)
  line L608 (1.467, 2.1411) -> (1.4683, 2.1265)
  line L609 (1.4683, 2.1265) -> (1.469, 2.1121)
  line L610 (1.469, 2.1121) -> (1.4692, 2.0978)
  line L611 (1.4692, 2.0978) -> (1.4689, 2.0837)
  line L612 (1.4689, 2.0837) -> (1.4679, 2.0698)
  line L613 (1.4679, 2.0698) -> (1.4672, 2.0629)
  line L614 (1.4672, 2.0629) -> (1.4668, 2.0595)
  line L615 (1.4668, 2.0595) -> (1.4663, 2.0562)
  line L616 (1.4663, 2.0562) -> (1.5187, 2.0344)
  line L617 (1.5187, 2.0344) -> (1.5208, 2.0372)
  line L618 (1.5208, 2.0372) -> (1.5229, 2.0399)
  line L619 (1.5229, 2.0399) -> (1.5272, 2.0452)
  line L620 (1.5272, 2.0452) -> (1.5364, 2.0557)
  line L621 (1.5364, 2.0557) -> (1.5461, 2.0659)
  line L622 (1.5461, 2.0659) -> (1.5563, 2.0759)
  line L623 (1.5563, 2.0759) -> (1.5671, 2.0856)
  line L624 (1.5671, 2.0856) -> (1.5783, 2.095)
  line L625 (1.5783, 2.095) -> (1.6251, 2.0711)
  line L626 (1.6251, 2.0711) -> (1.6241, 2.0566)
  line L627 (1.6241, 2.0566) -> (1.6225, 2.0422)
  line L628 (1.6225, 2.0422) -> (1.6205, 2.028)
  line L629 (1.6205, 2.028) -> (1.6179, 2.0142)
  line L630 (1.6179, 2.0142) -> (1.6149, 2.0006)
  line L631 (1.6149, 2.0006) -> (1.6131, 1.9939)
  line L632 (1.6131, 1.9939) -> (1.6121, 1.9906)
  line L633 (1.6121, 1.9906) -> (1.6111, 1.9874)
  line L634 (1.6111, 1.9874) -> (1.6595, 1.9577)
  line L635 (1.6595, 1.9577) -> (1.662, 1.9601)
  line L636 (1.662, 1.9601) -> (1.6645, 1.9624)
  line L637 (1.6645, 1.9624) -> (1.6696, 1.9671)
  line L638 (1.6696, 1.9671) -> (1.6803, 1.976)
  line L639 (1.6803, 1.976) -> (1.6915, 1.9846)
  line L640 (1.6915, 1.9846) -> (1.7031, 1.9928)
  line L641 (1.7031, 1.9928) -> (1.7153, 2.0007)
  line L642 (1.7153, 2.0007) -> (1.7278, 2.0083)
  line L643 (1.7278, 2.0083) -> (1.7703, 1.9773)
  line L644 (1.7703, 1.9773) -> (1.767, 1.9631)
  line L645 (1.767, 1.9631) -> (1.7632, 1.9491)
  line L646 (1.7632, 1.9491) -> (1.759, 1.9355)
  line L647 (1.759, 1.9355) -> (1.7543, 1.9222)
  line L648 (1.7543, 1.9222) -> (1.7491, 1.9093)
  line L649 (1.7491, 1.9093) -> (1.7463, 1.903)
  line L650 (1.7463, 1.903) -> (1.7449, 1.8999)
  line L651 (1.7449, 1.8999) -> (1.7434, 1.8968)
  line L652 (1.7434, 1.8968) -> (1.7865, 1.8599)
  line L653 (1.7865, 1.8599) -> (1.7893, 1.8619)
  line L654 (1.7893, 1.8619) -> (1.7922, 1.8638)
  line L655 (1.7922, 1.8638) -> (1.798, 1.8676)
  line L656 (1.798, 1.8676) -> (1.8099, 1.8747)
  line L657 (1.8099, 1.8747) -> (1.8223, 1.8814)
  line L658 (1.8223, 1.8814) -> (1.8351, 1.8877)
  line L659 (1.8351, 1.8877) -> (1.8483, 1.8936)
  line L660 (1.8483, 1.8936) -> (1.8619, 1.8992)
  line L661 (1.8619, 1.8992) -> (1.8991, 1.862)
  line L662 (1.8991, 1.862) -> (1.8936, 1.8484)
  line L663 (1.8936, 1.8484) -> (1.8877, 1.8352)
  line L664 (1.8877, 1.8352) -> (1.8814, 1.8224)
  line L665 (1.8814, 1.8224) -> (1.8747, 1.81)
  line L666 (1.8747, 1.81) -> (1.8675, 1.798)
  line L667 (1.8675, 1.798) -> (1.8637, 1.7923)
  line L668 (1.8637, 1.7923) -> (1.8618, 1.7894)
  line L669 (1.8618, 1.7894) -> (1.8599, 1.7866)
  line L670 (1.8599, 1.7866) -> (1.8967, 1.7435)
  line L671 (1.8967, 1.7435) -> (1.8998, 1.745)
  line L672 (1.8998, 1.745) -> (1.9029, 1.7464)
  line L673 (1.9029, 1.7464) -> (1.9092, 1.7492)
  line L674 (1.9092, 1.7492) -> (1.9221, 1.7544)
  line L675 (1.9221, 1.7544) -> (1.9354, 1.7591)
  line L676 (1.9354, 1.7591) -> (1.9491, 1.7633)
  line L677 (1.9491, 1.7633) -> (1.963, 1.7671)
  line L678 (1.963, 1.7671) -> (1.9773, 1.7704)
  line L679 (1.9773, 1.7704) -> (2.0082, 1.7279)
  line L680 (2.0082, 1.7279) -> (2.0006, 1.7153)
  line L681 (2.0006, 1.7153) -> (1.9927, 1.7032)
  line L682 (1.9927, 1.7032) -> (1.9845, 1.6916)
  line L683 (1.9845, 1.6916) -> (1.9759, 1.6804)
  line L684 (1.9759, 1.6804) -> (1.967, 1.6697)
  line L685 (1.967, 1.6697) -> (1.9624, 1.6645)
  line L686 (1.9624, 1.6645) -> (1.96, 1.662)
  line L687 (1.96, 1.662) -> (1.9577, 1.6596)
  line L688 (1.9577, 1.6596) -> (1.9873, 1.6112)
  line L689 (1.9873, 1.6112) -> (1.9906, 1.6122)
  line L690 (1.9906, 1.6122) -> (1.9939, 1.6132)
  line L691 (1.9939, 1.6132) -> (2.0005, 1.6149)
  line L692 (2.0005, 1.6149) -> (2.0141, 1.618)
  line L693 (2.0141, 1.618) -> (2.028, 1.6206)
  line L694 (2.028, 1.6206) -> (2.0421, 1.6226)
  line L695 (2.0421, 1.6226) -> (2.0565, 1.6242)
  line L696 (2.0565, 1.6242) -> (2.0711, 1.6252)
  line L697 (2.0711, 1.6252) -> (2.095, 1.5783)
  line L698 (2.095, 1.5783) -> (2.0855, 1.5672)
  line L699 (2.0855, 1.5672) -> (2.0758, 1.5564)
  line L700 (2.0758, 1.5564) -> (2.0659, 1.5462)
  line L701 (2.0659, 1.5462) -> (2.0557, 1.5365)
  line L702 (2.0557, 1.5365) -> (2.0452, 1.5273)
  line L703 (2.0452, 1.5273) -> (2.0398, 1.523)
  line L704 (2.0398, 1.523) -> (2.0371, 1.5209)
  line L705 (2.0371, 1.5209) -> (2.0344, 1.5188)
  line L706 (2.0344, 1.5188) -> (2.0561, 1.4664)
  line L707 (2.0561, 1.4664) -> (2.0595, 1.4669)
  line L708 (2.0595, 1.4669) -> (2.0629, 1.4673)
  line L709 (2.0629, 1.4673) -> (2.0697, 1.468)
  line L710 (2.0697, 1.468) -> (2.0836, 1.469)
  line L711 (2.0836, 1.469) -> (2.0977, 1.4693)
  line L712 (2.0977, 1.4693) -> (2.112, 1.4691)
  line L713 (2.112, 1.4691) -> (2.1265, 1.4684)
  line L714 (2.1265, 1.4684) -> (2.141, 1.4671)
  line L715 (2.141, 1.4671) -> (2.1573, 1.4171)
  line L716 (2.1573, 1.4171) -> (2.1462, 1.4075)
  line L717 (2.1462, 1.4075) -> (2.135, 1.3984)
  line L718 (2.135, 1.3984) -> (2.1235, 1.3899)
  line L719 (2.1235, 1.3899) -> (2.1119, 1.3819)
  line L720 (2.1119, 1.3819) -> (2.1001, 1.3745)
  line L721 (2.1001, 1.3745) -> (2.0942, 1.371)
  line L722 (2.0942, 1.371) -> (2.0912, 1.3694)
  line L723 (2.0912, 1.3694) -> (2.0881, 1.3678)
  line L724 (2.0881, 1.3678) -> (2.1014, 1.3126)
  line L725 (2.1014, 1.3126) -> (2.1048, 1.3125)
  line L726 (2.1048, 1.3125) -> (2.1082, 1.3124)
  line L727 (2.1082, 1.3124) -> (2.1151, 1.3121)
  line L728 (2.1151, 1.3121) -> (2.129, 1.3108)
  line L729 (2.129, 1.3108) -> (2.143, 1.3089)
  line L730 (2.143, 1.3089) -> (2.157, 1.3065)
  line L731 (2.157, 1.3065) -> (2.1712, 1.3035)
  line L732 (2.1712, 1.3035) -> (2.1854, 1.3)
  line L733 (2.1854, 1.3) -> (2.1936, 1.2482)
  line L734 (2.1936, 1.2482) -> (2.1812, 1.2405)
  line L735 (2.1812, 1.2405) -> (2.1687, 1.2333)
  line L736 (2.1687, 1.2333) -> (2.156, 1.2266)
  line L737 (2.156, 1.2266) -> (2.1433, 1.2205)
  line L738 (2.1433, 1.2205) -> (2.1305, 1.2151)
  line L739 (2.1305, 1.2151) -> (2.1241, 1.2126)
  line L740 (2.1241, 1.2126) -> (2.1208, 1.2114)
  line L741 (2.1208, 1.2114) -> (2.1176, 1.2103)
  line L742 (2.1176, 1.2103) -> (2.122, 1.1538)
  line L743 (2.122, 1.1538) -> (2.1254, 1.1532)
  point P0 (0, 0)
  constraints: 1488 end point, 298 perpendicular, 50 parallel
extrude "Extrusion1" add sketch "Sketch1" along normal blind 0.3